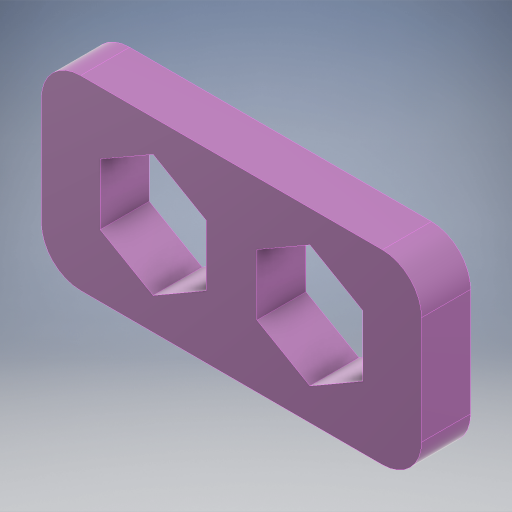
# Autodesk Inventor part: М3x2 вставка
Saved by Autodesk Inventor 2023 (Build 270158000, 158)
## iProperties
Created: 2023-03-26
Part Number: М3x2 вставка
Material: Типовые
Document SubType Name: Modeling
Designer: Admin
Density: 1 g/cm^3
Appearance: По умолчанию
Author: Admin
Autodesk Inventor part; units mm, degrees
ref_plane "YZ Plane" through (0, 0, 0) normal (1, 0, 0) x (0, 1, 0)
ref_plane "XZ Plane" through (0, 0, 0) normal (0, 1, 0) x (-1, 0, 0)
ref_plane "XY Plane" through (0, 0, 0) normal (0, 0, 1) x (1, 0, 0)
sketch "Эскиз1" plane through (0, 0, 0) normal (0, 0, 1) x (1, 0, 0)
  circle A0 centre (-4, 0) radius 1.5
  circle A1 centre (4, 0) radius 1.5
  arc A2 (-9.7, -2.75) -> (-7.7, -4.75) centre (-7.7, -2.75) ccw
  line L0 (6.7, -1.5588) -> (4, -3.1177)
  line L1 (6.7, 1.5588) -> (6.7, -1.5588)
  line L2 (-7.7, -4.75) -> (7.7, -4.75)
  line L3 (9.7, -2.75) -> (9.7, 2.75)
  line L4 (4, -3.1177) -> (1.3, -1.5588)
  line L5 (4, 3.1177) -> (6.7, 1.5588)
  arc A3 (9.7, 2.75) -> (7.7, 4.75) centre (7.7, 2.75) ccw
  line L6 (1.3, -1.5588) -> (1.3, 1.5588)
  line L7 (-9.7, 2.75) -> (-9.7, -2.75)
  line L8 (1.3, 1.5588) -> (4, 3.1177)
  arc A4 (-7.7, 4.75) -> (-9.7, 2.75) centre (-7.7, 2.75) ccw
  line L9 (7.7, 4.75) -> (-7.7, 4.75)
  arc A5 (7.7, -4.75) -> (9.7, -2.75) centre (7.7, -2.75) ccw
  line L10 (0, -4.75) -> (0, 36.1208) construction
  line L11 (-4, 3.1177) -> (-6.7, 1.5588)
  line L12 (-6.7, -1.5588) -> (-4, -3.1177)
  line L13 (-6.7, 1.5588) -> (-6.7, -1.5588)
  line L14 (-1.3, -1.5588) -> (-1.3, 1.5588)
  line L15 (-4, -3.1177) -> (-1.3, -1.5588)
  line L16 (-1.3, 1.5588) -> (-4, 3.1177)
  point P0 (0, 0)
  point P1 (6.7, 0)
  point P2 (9.7, 0)
  dimension "d1" = 2
  dimension "d2" = 2
  dimension "d7" = 3
  dimension "d8" = 4
  constraints: 34 end point, 8 point on circle, 8 tangent, 7 symmetric about line, 6 centre point, 4 parallel, 3 equal radius, 3 horizontal alignment, 3 midpoint, 2 coincident, 2 vertical, 1 horizontal, 1 perpendicular, 1 vertical alignment, 13 other
  measures "d1" radius of A4
  measures "d2" radius of A5
  measures "d7" diameter of A1
  measures "d8" distance of point (0, 0) point (4, 0)
extrude "Выдавливание1" add sketch "Эскиз1" along normal blind 2.5 contours L7 A4 L9 A3 L3 A5 L2 A2
